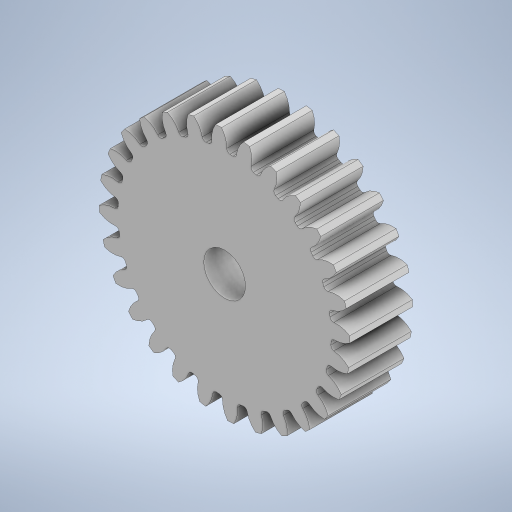
# Autodesk Inventor part: Spur_Gear_28
Saved by Autodesk Inventor 2024 (Build 280153000, 153)
## iProperties
Created: 2024-10-21
Part Number: Spur_Gear_28
Material: Generic
Document SubType Name: Modeling
Designer: Yash Purswani
Density: 1 g/cm^3
Appearance: Default
Author: Yash Purswani
Autodesk Inventor part; units mm, degrees
ref_plane "YZ Plane" through (0, 0, 0) normal (1, 0, 0) x (0, 1, 0)
ref_plane "XZ Plane" through (0, 0, 0) normal (0, 1, 0) x (-1, 0, 0)
ref_plane "XY Plane" through (0, 0, 0) normal (0, 0, 1) x (1, 0, 0)
sketch "Sketch1" plane through (0, 0, 0) normal (0, 0, 1) x (1, 0, 0)
  circle A0 centre (0, 0) radius 28 construction
  line L0 (0, 30) -> (0, 28.77)
  arc A1 (0.5033, 26.2967) -> (-0.7297, 29.9911) centre (-5.3709, 26.3891) ccw
  arc A2 (0.5033, 26.2967) -> (1.2646, 25.4686) centre (1.3044, 26.2691) ccw
  arc A3 (-2.1783, 29.9208) -> (-3.056, 26.1234) centre (2.6898, 26.7954) ccw
  arc A4 (-3.7332, 25.2252) -> (-3.056, 26.1234) centre (-3.8506, 26.0181) ccw
  arc A5 (-8.7816, 28.6859) -> (-8.7924, 24.7884) centre (-3.3402, 26.7222) ccw
  arc A6 (-5.3608, 25.7494) -> (-7.3851, 29.0768) centre (-11.1084, 24.5323) ccw
  arc A7 (-9.2528, 23.7621) -> (-8.7924, 24.7884) centre (-9.5436, 24.509) ccw
  arc A8 (-5.3608, 25.7494) -> (-4.4344, 25.1115) centre (-4.5737, 25.9008) ccw
  arc A9 (-14.9447, 26.0126) -> (-14.0879, 22.2104) centre (-9.2027, 25.3089) ccw
  arc A10 (-10.9562, 23.9109) -> (-13.6701, 26.7045) centre (-16.2888, 21.4454) ccw
  arc A11 (-14.3084, 21.1074) -> (-14.0879, 22.2104) centre (-14.7581, 21.7708) ccw
  arc A12 (-10.9562, 23.9109) -> (-9.911, 23.4951) centre (-10.2225, 24.2336) ccw
  arc A13 (-20.3584, 22.0349) -> (-18.6769, 18.5187) centre (-14.6037, 22.6266) ccw
  arc A14 (-16.0022, 20.8734) -> (-19.2697, 22.993) centre (-20.6525, 17.2831) ccw
  arc A15 (-18.6464, 17.3943) -> (-18.6769, 18.5187) centre (-19.2325, 17.941) ccw
  arc A16 (-16.0022, 20.8734) -> (-14.8907, 20.7007) centre (-15.3587, 21.3513) ccw
  arc A17 (-24.7512, 16.9523) -> (-22.3295, 13.8984) centre (-19.2724, 18.8097) ccw
  arc A18 (-20.2458, 16.7893) -> (-23.903, 18.1286) centre (-23.9805, 12.2542) ccw
  arc A19 (-22.0495, 12.8089) -> (-22.3295, 13.8984) centre (-22.7426, 13.2115) ccw
  arc A20 (-20.2458, 16.7893) -> (-19.1237, 16.8682) centre (-19.7248, 17.3984) ccw
  arc A21 (-27.9028, 11.0196) -> (-24.8623, 8.5811) centre (-22.9748, 14.0495) ccw
  arc A22 (-23.4741, 11.8632) -> (-27.3377, 12.3552) centre (-26.1061, 6.6108) ccw
  arc A23 (-24.347, 7.5813) -> (-24.8623, 8.5811) centre (-25.1122, 7.8196) ccw
  arc A24 (-23.4741, 11.8632) -> (-22.3977, 12.1898) centre (-23.1017, 12.573) ccw
  arc A25 (-29.6553, 4.5344) -> (-26.1484, 2.8336) centre (-25.5251, 8.5849) ccw
  arc A26 (-25.5254, 6.3423) -> (-29.4016, 5.9622) centre (-26.9226, 0.6359) ccw
  arc A27 (-25.4235, 1.9735) -> (-26.1484, 2.8336) centre (-26.2226, 2.0355) ccw
  arc A28 (-25.5254, 6.3423) -> (-24.5487, 6.9002) centre (-25.3203, 7.1171) ccw
  arc A29 (-29.9208, -2.1783) -> (-26.1234, -3.056) centre (-26.7954, 2.6898) ccw
  arc A30 (-26.2967, 0.5033) -> (-29.9911, -0.7297) centre (-26.3891, -5.3709) ccw
  arc A31 (-25.2252, -3.7332) -> (-26.1234, -3.056) centre (-26.0181, -3.8506) ccw
  arc A32 (-26.2967, 0.5033) -> (-25.4686, 1.2646) centre (-26.2691, 1.3044) ccw
  arc A33 (-28.6859, -8.7816) -> (-24.7884, -8.7924) centre (-26.7222, -3.3402) ccw
  arc A34 (-25.7494, -5.3608) -> (-29.0768, -7.3851) centre (-24.5323, -11.1084) ccw
  arc A35 (-23.7621, -9.2528) -> (-24.7884, -8.7924) centre (-24.509, -9.5436) ccw
  arc A36 (-25.7494, -5.3608) -> (-25.1115, -4.4344) centre (-25.9008, -4.5737) ccw
  arc A37 (-26.0126, -14.9447) -> (-22.2104, -14.0879) centre (-25.3089, -9.2027) ccw
  arc A38 (-23.9109, -10.9562) -> (-26.7045, -13.6701) centre (-21.4454, -16.2888) ccw
  arc A39 (-21.1074, -14.3084) -> (-22.2104, -14.0879) centre (-21.7708, -14.7581) ccw
  arc A40 (-23.9109, -10.9562) -> (-23.4951, -9.911) centre (-24.2336, -10.2225) ccw
  arc A41 (-22.0349, -20.3584) -> (-18.5187, -18.6769) centre (-22.6266, -14.6037) ccw
  arc A42 (-20.8734, -16.0022) -> (-22.993, -19.2697) centre (-17.2831, -20.6525) ccw
  arc A43 (-17.3943, -18.6464) -> (-18.5187, -18.6769) centre (-17.941, -19.2325) ccw
  arc A44 (-20.8734, -16.0022) -> (-20.7007, -14.8907) centre (-21.3513, -15.3587) ccw
  arc A45 (-16.9523, -24.7512) -> (-13.8984, -22.3295) centre (-18.8097, -19.2724) ccw
  arc A46 (-16.7893, -20.2458) -> (-18.1286, -23.903) centre (-12.2542, -23.9805) ccw
  arc A47 (-12.8089, -22.0495) -> (-13.8984, -22.3295) centre (-13.2115, -22.7426) ccw
  arc A48 (-16.7893, -20.2458) -> (-16.8682, -19.1237) centre (-17.3984, -19.7248) ccw
  arc A49 (-11.0196, -27.9028) -> (-8.5811, -24.8623) centre (-14.0495, -22.9748) ccw
  arc A50 (-11.8632, -23.4741) -> (-12.3552, -27.3377) centre (-6.6108, -26.1061) ccw
  arc A51 (-7.5813, -24.347) -> (-8.5811, -24.8623) centre (-7.8196, -25.1122) ccw
  arc A52 (-11.8632, -23.4741) -> (-12.1898, -22.3977) centre (-12.573, -23.1017) ccw
  arc A53 (-4.5344, -29.6553) -> (-2.8336, -26.1484) centre (-8.5849, -25.5251) ccw
  arc A54 (-6.3423, -25.5254) -> (-5.9622, -29.4016) centre (-0.6359, -26.9226) ccw
  arc A55 (-1.9735, -25.4235) -> (-2.8336, -26.1484) centre (-2.0355, -26.2226) ccw
  arc A56 (-6.3423, -25.5254) -> (-6.9002, -24.5487) centre (-7.1171, -25.3203) ccw
  arc A57 (2.1783, -29.9208) -> (3.056, -26.1234) centre (-2.6898, -26.7954) ccw
  arc A58 (-0.5033, -26.2967) -> (0.7297, -29.9911) centre (5.3709, -26.3891) ccw
  arc A59 (3.7332, -25.2252) -> (3.056, -26.1234) centre (3.8506, -26.0181) ccw
  arc A60 (-0.5033, -26.2967) -> (-1.2646, -25.4686) centre (-1.3044, -26.2691) ccw
  arc A61 (8.7816, -28.6859) -> (8.7924, -24.7884) centre (3.3402, -26.7222) ccw
  arc A62 (5.3608, -25.7494) -> (7.3851, -29.0768) centre (11.1084, -24.5323) ccw
  arc A63 (9.2528, -23.7621) -> (8.7924, -24.7884) centre (9.5436, -24.509) ccw
  arc A64 (5.3608, -25.7494) -> (4.4344, -25.1115) centre (4.5737, -25.9008) ccw
  arc A65 (14.9447, -26.0126) -> (14.0879, -22.2104) centre (9.2027, -25.3089) ccw
  arc A66 (10.9562, -23.9109) -> (13.6701, -26.7045) centre (16.2888, -21.4454) ccw
  arc A67 (14.3084, -21.1074) -> (14.0879, -22.2104) centre (14.7581, -21.7708) ccw
  arc A68 (10.9562, -23.9109) -> (9.911, -23.4951) centre (10.2225, -24.2336) ccw
  arc A69 (20.3584, -22.0349) -> (18.6769, -18.5187) centre (14.6037, -22.6266) ccw
  arc A70 (16.0022, -20.8734) -> (19.2697, -22.993) centre (20.6525, -17.2831) ccw
  arc A71 (18.6464, -17.3943) -> (18.6769, -18.5187) centre (19.2325, -17.941) ccw
  arc A72 (16.0022, -20.8734) -> (14.8907, -20.7007) centre (15.3587, -21.3513) ccw
  arc A73 (24.7512, -16.9523) -> (22.3295, -13.8984) centre (19.2724, -18.8097) ccw
  arc A74 (20.2458, -16.7893) -> (23.903, -18.1286) centre (23.9805, -12.2542) ccw
  arc A75 (22.0495, -12.8089) -> (22.3295, -13.8984) centre (22.7426, -13.2115) ccw
  arc A76 (20.2458, -16.7893) -> (19.1237, -16.8682) centre (19.7248, -17.3984) ccw
  arc A77 (27.9028, -11.0196) -> (24.8623, -8.5811) centre (22.9748, -14.0495) ccw
  arc A78 (23.4741, -11.8632) -> (27.3377, -12.3552) centre (26.1061, -6.6108) ccw
  arc A79 (24.347, -7.5813) -> (24.8623, -8.5811) centre (25.1122, -7.8196) ccw
  arc A80 (23.4741, -11.8632) -> (22.3977, -12.1898) centre (23.1017, -12.573) ccw
  arc A81 (29.6553, -4.5344) -> (26.1484, -2.8336) centre (25.5251, -8.5849) ccw
  arc A82 (25.5254, -6.3423) -> (29.4016, -5.9622) centre (26.9226, -0.6359) ccw
  arc A83 (25.4235, -1.9735) -> (26.1484, -2.8336) centre (26.2226, -2.0355) ccw
  arc A84 (25.5254, -6.3423) -> (24.5487, -6.9002) centre (25.3203, -7.1171) ccw
  arc A85 (29.9208, 2.1783) -> (26.1234, 3.056) centre (26.7954, -2.6898) ccw
  arc A86 (26.2967, -0.5033) -> (29.9911, 0.7297) centre (26.3891, 5.3709) ccw
  arc A87 (25.2252, 3.7332) -> (26.1234, 3.056) centre (26.0181, 3.8506) ccw
  arc A88 (26.2967, -0.5033) -> (25.4686, -1.2646) centre (26.2691, -1.3044) ccw
  arc A89 (28.6859, 8.7816) -> (24.7884, 8.7924) centre (26.7222, 3.3402) ccw
  arc A90 (25.7494, 5.3608) -> (29.0768, 7.3851) centre (24.5323, 11.1084) ccw
  arc A91 (23.7621, 9.2528) -> (24.7884, 8.7924) centre (24.509, 9.5436) ccw
  arc A92 (25.7494, 5.3608) -> (25.1115, 4.4344) centre (25.9008, 4.5737) ccw
  arc A93 (26.0126, 14.9447) -> (22.2104, 14.0879) centre (25.3089, 9.2027) ccw
  arc A94 (23.9109, 10.9562) -> (26.7045, 13.6701) centre (21.4454, 16.2888) ccw
  arc A95 (21.1074, 14.3084) -> (22.2104, 14.0879) centre (21.7708, 14.7581) ccw
  arc A96 (23.9109, 10.9562) -> (23.4951, 9.911) centre (24.2336, 10.2225) ccw
  arc A97 (22.0349, 20.3584) -> (18.5187, 18.6769) centre (22.6266, 14.6037) ccw
  arc A98 (20.8734, 16.0022) -> (22.993, 19.2697) centre (17.2831, 20.6525) ccw
  arc A99 (17.3943, 18.6464) -> (18.5187, 18.6769) centre (17.941, 19.2325) ccw
  arc A100 (20.8734, 16.0022) -> (20.7007, 14.8907) centre (21.3513, 15.3587) ccw
  arc A101 (16.9523, 24.7512) -> (13.8984, 22.3295) centre (18.8097, 19.2724) ccw
  arc A102 (16.7893, 20.2458) -> (18.1286, 23.903) centre (12.2542, 23.9805) ccw
  arc A103 (12.8089, 22.0495) -> (13.8984, 22.3295) centre (13.2115, 22.7426) ccw
  arc A104 (16.7893, 20.2458) -> (16.8682, 19.1237) centre (17.3984, 19.7248) ccw
  arc A105 (11.0196, 27.9028) -> (8.5811, 24.8623) centre (14.0495, 22.9748) ccw
  arc A106 (11.8632, 23.4741) -> (12.3552, 27.3377) centre (6.6108, 26.1061) ccw
  arc A107 (7.5813, 24.347) -> (8.5811, 24.8623) centre (7.8196, 25.1122) ccw
  arc A108 (11.8632, 23.4741) -> (12.1898, 22.3977) centre (12.573, 23.1017) ccw
  arc A109 (4.5344, 29.6553) -> (2.8336, 26.1484) centre (8.5849, 25.5251) ccw
  arc A110 (6.3423, 25.5254) -> (5.9622, 29.4016) centre (0.6359, 26.9226) ccw
  arc A111 (1.9735, 25.4235) -> (2.8336, 26.1484) centre (2.0355, 26.2226) ccw
  arc A112 (6.3423, 25.5254) -> (6.9002, 24.5487) centre (7.1171, 25.3203) ccw
  arc A113 (-7.3851, 29.0768) -> (-8.7816, 28.6859) centre (0, 0) ccw
  arc A114 (-0.7297, 29.9911) -> (-2.1783, 29.9208) centre (0, 0) ccw
  arc A115 (5.9622, 29.4016) -> (4.5344, 29.6553) centre (0, 0) ccw
  arc A116 (12.3552, 27.3377) -> (11.0196, 27.9028) centre (0, 0) ccw
  arc A117 (22.993, 19.2697) -> (22.0349, 20.3584) centre (0, 0) ccw
  arc A118 (18.1286, 23.903) -> (16.9523, 24.7512) centre (0, 0) ccw
  arc A119 (26.7045, 13.6701) -> (26.0126, 14.9447) centre (0, 0) ccw
  arc A120 (29.0768, 7.3851) -> (28.6859, 8.7816) centre (0, 0) ccw
  arc A121 (29.9911, 0.7297) -> (29.9208, 2.1783) centre (0, 0) ccw
  arc A122 (29.4016, -5.9622) -> (29.6553, -4.5344) centre (0, 0) ccw
  arc A123 (27.3377, -12.3552) -> (27.9028, -11.0196) centre (0, 0) ccw
  arc A124 (23.903, -18.1286) -> (24.7512, -16.9523) centre (0, 0) ccw
  arc A125 (19.2697, -22.993) -> (20.3584, -22.0349) centre (0, 0) ccw
  arc A126 (13.6701, -26.7045) -> (14.9447, -26.0126) centre (0, 0) ccw
  arc A127 (7.3851, -29.0768) -> (8.7816, -28.6859) centre (0, 0) ccw
  arc A128 (0.7297, -29.9911) -> (2.1783, -29.9208) centre (0, 0) ccw
  arc A129 (-5.9622, -29.4016) -> (-4.5344, -29.6553) centre (0, 0) ccw
  arc A130 (-12.3552, -27.3377) -> (-11.0196, -27.9028) centre (0, 0) ccw
  arc A131 (-18.1286, -23.903) -> (-16.9523, -24.7512) centre (0, 0) ccw
  arc A132 (-22.993, -19.2697) -> (-22.0349, -20.3584) centre (0, 0) ccw
  arc A133 (-26.7045, -13.6701) -> (-26.0126, -14.9447) centre (0, 0) ccw
  arc A134 (-29.0768, -7.3851) -> (-28.6859, -8.7816) centre (0, 0) ccw
  arc A135 (-29.9911, -0.7297) -> (-29.9208, -2.1783) centre (0, 0) ccw
  arc A136 (-29.4016, 5.9622) -> (-29.6553, 4.5344) centre (0, 0) ccw
  arc A137 (-27.3377, 12.3552) -> (-27.9028, 11.0196) centre (0, 0) ccw
  arc A138 (-23.903, 18.1286) -> (-24.7512, 16.9523) centre (0, 0) ccw
  arc A139 (-13.6701, 26.7045) -> (-14.9447, 26.0126) centre (0, 0) ccw
  arc A140 (-19.2697, 22.993) -> (-20.3584, 22.0349) centre (0, 0) ccw
  arc A141 (-3.7332, 25.2252) -> (-4.4344, 25.1115) centre (0, 0) ccw
  arc A142 (1.9735, 25.4235) -> (1.2646, 25.4686) centre (0, 0) ccw
  arc A143 (7.5813, 24.347) -> (6.9002, 24.5487) centre (0, 0) ccw
  arc A144 (12.8089, 22.0495) -> (12.1898, 22.3977) centre (0, 0) ccw
  arc A145 (-9.2528, 23.7621) -> (-9.911, 23.4951) centre (0, 0) ccw
  arc A146 (-14.3084, 21.1074) -> (-14.8907, 20.7007) centre (0, 0) ccw
  arc A147 (-18.6464, 17.3943) -> (-19.1237, 16.8682) centre (0, 0) ccw
  arc A148 (-23.7621, -9.2528) -> (-23.4951, -9.911) centre (0, 0) ccw
  arc A149 (-21.1074, -14.3084) -> (-20.7007, -14.8907) centre (0, 0) ccw
  arc A150 (-7.5813, -24.347) -> (-6.9002, -24.5487) centre (0, 0) ccw
  arc A151 (-17.3943, -18.6464) -> (-16.8682, -19.1237) centre (0, 0) ccw
  arc A152 (-12.8089, -22.0495) -> (-12.1898, -22.3977) centre (0, 0) ccw
  arc A153 (-1.9735, -25.4235) -> (-1.2646, -25.4686) centre (0, 0) ccw
  arc A154 (3.7332, -25.2252) -> (4.4344, -25.1115) centre (0, 0) ccw
  arc A155 (9.2528, -23.7621) -> (9.911, -23.4951) centre (0, 0) ccw
  arc A156 (14.3084, -21.1074) -> (14.8907, -20.7007) centre (0, 0) ccw
  arc A157 (18.6464, -17.3943) -> (19.1237, -16.8682) centre (0, 0) ccw
  arc A158 (22.0495, -12.8089) -> (22.3977, -12.1898) centre (0, 0) ccw
  arc A159 (23.7621, 9.2528) -> (23.4951, 9.911) centre (0, 0) ccw
  arc A160 (25.2252, 3.7332) -> (25.1115, 4.4344) centre (0, 0) ccw
  arc A161 (24.347, -7.5813) -> (24.5487, -6.9002) centre (0, 0) ccw
  arc A162 (25.4235, -1.9735) -> (25.4686, -1.2646) centre (0, 0) ccw
  arc A163 (21.1074, 14.3084) -> (20.7007, 14.8907) centre (0, 0) ccw
  arc A164 (17.3943, 18.6464) -> (16.8682, 19.1237) centre (0, 0) ccw
  arc A165 (-22.0495, 12.8089) -> (-22.3977, 12.1898) centre (0, 0) ccw
  arc A166 (-24.347, 7.5813) -> (-24.5487, 6.9002) centre (0, 0) ccw
  arc A167 (-25.4235, 1.9735) -> (-25.4686, 1.2646) centre (0, 0) ccw
  arc A168 (-25.2252, -3.7332) -> (-25.1115, -4.4344) centre (0, 0) ccw
  circle A169 centre (0, 0) radius 5
  point P0 (-6.4019, 28.0487)
  point P1 (-12.4828, 25.9209)
  point P2 (-17.9378, 22.4933)
  point P3 (-22.4933, 17.9378)
  point P4 (-25.9209, 12.4828)
  point P5 (-28.0487, 6.4019)
  point P6 (-28.77, 0)
  point P7 (-28.0487, -6.4019)
  point P8 (-25.9209, -12.4828)
  point P9 (-22.4933, -17.9378)
  point P10 (-17.9378, -22.4933)
  point P11 (-12.4828, -25.9209)
  point P12 (-6.4019, -28.0487)
  point P13 (0, -28.77)
  point P14 (6.4019, -28.0487)
  point P15 (12.4828, -25.9209)
  point P16 (17.9378, -22.4933)
  point P17 (22.4933, -17.9378)
  point P18 (25.9209, -12.4828)
  point P19 (28.0487, -6.4019)
  point P20 (28.77, 0)
  point P21 (28.0487, 6.4019)
  point P22 (25.9209, 12.4828)
  point P23 (22.4933, 17.9378)
  point P24 (17.9378, 22.4933)
  point P25 (12.4828, 25.9209)
  point P26 (6.4019, 28.0487)
  point P27 (0, 5)
  dimension "d24" = 10
  dimension "d1" = 56
  dimension "d13" = 360
  constraints: 252 point on circle, 113 centre point, 3 coincident, 2 end point, 1 point on line, 1 vertical, 1 vertical alignment, 620 other
  measures "d1" diameter of A0
extrude "Extrusion1" add sketch "Sketch1" along normal blind 15
body "Solid1"
